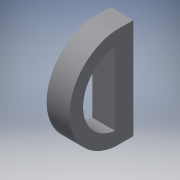
# Autodesk Inventor part: hook_loop
Saved by Autodesk Inventor 2016 (Build 200138000, 138)
## iProperties
Created: 2016-06-23
Part Number: hook_loop
Material: Generic
Document SubType Name: Modeling
Designer: ajar021
Density: 1 g/cm^3
Appearance: Default
Author: ajar021
Autodesk Inventor part; units mm, degrees
ref_plane "YZ Plane" through (0, 0, 0) normal (1, 0, 0) x (0, 1, 0)
ref_plane "XZ Plane" through (0, 0, 0) normal (0, 1, 0) x (-1, 0, 0)
ref_plane "XY Plane" through (0, 0, 0) normal (0, 0, 1) x (1, 0, 0)
sketch "Sketch1" plane through (0, 0, 0) normal (0, 0, 1) x (1, 0, 0)
  circle A0 centre (1.9343, 0.0365) radius 1.25 construction
  line L0 (0.6843, -5.4635) -> (3.1843, -5.4635)
  line L1 (3.1843, -5.4635) -> (3.1843, 5.5365)
  line L2 (3.1843, 5.5365) -> (0.6843, 5.5365)
  line L3 (0.6843, 5.5365) -> (0.6843, -5.4635)
  line L4 (0.6843, -5.4635) -> (3.1843, 5.5365) construction
  line L5 (3.1843, -5.4635) -> (0.6843, 5.5365) construction
  point P0 (0, 0)
  dimension "d0" = 11
  dimension "d1" = 2.5
  constraints: 12 end point, 2 midpoint, 2 parallel, 1 horizontal, 1 perpendicular
  measures "d0" distance of L2.end L0.start
  measures "d1" distance of L0.start L0.end
extrude "Extrusion1" add sketch "Sketch1" along normal blind 2
sketch "Sketch2" plane through (3.1843, -5.4635, 0) normal (1, 0, 0) x (0, 0, -1)
  line L0 (-2, 0) -> (-2, 11) projected
  line L1 (-2, 0) -> (-2, 11)
  line L2 (-2, 5.5) -> (-7, 5.5)
  arc A0 (-2, 11) -> (-2, 0) centre (-1.475, 5.5) ccw
  line L3 (-2, 0) -> (-2, 1.5)
  line L4 (-2, 11) -> (-2, 9.5)
  line L5 (-7, 5.5) -> (-5.5, 5.5)
  arc A1 (-2, 9.5) -> (-2, 1.5) centre (-1.475, 5.5) ccw
  point P0 (0, 5.4635)
  dimension "d4" = 5
  dimension "d5" = 1.5
  dimension "d6" = 1.5
  dimension "d7" = 1.5
  constraints: 10 end point, 5 point on circle, 3 point on line, 2 centre point, 1 collinear, 1 horizontal, 1 midpoint
  measures "d4" distance of L2.start L2.end
  measures "d5" distance of L0.start L3.end
  measures "d6" distance of L0.end L4.end
  measures "d7" distance of L2.end L5.end
extrude "Extrusion2" add sketch "Sketch2" against normal up to surface (2.5 mm away) contours A0 L2 A1 L0 | A0 L0 A1 L2
equation "\"d6\" = d5"
equation "\"d7\" = d5"
body "Solid1"
